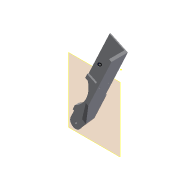
# Autodesk Inventor part: 30_CUBE_openSIM_Laserarm_532nm
Saved by Autodesk Inventor 2019 (Build 230136000, 136)
## iProperties
Created: 2019-08-28
Part Number: 30_CUBE_openSIM_Laserarm_532nm
Material: Generic
Document SubType Name: Modeling
Designer: diederichbenedict
Density: 1 g/cm^3
Appearance: Default
Author: diederichbenedict
Autodesk Inventor part; units mm, degrees
ref_plane "YZ Plane" through (0, 0, 0) normal (1, 0, 0) x (0, 1, 0)
ref_plane "Work Plane1" through (0, 0, 0) normal (0, 0, 1) x (1, 0, 0)
ref_plane "Work Plane3" through (52.5471, 38.1824, 4.95) normal (0, 0, -1) x (0, 1, 0)
sketch "Sketch1" plane through (0, 0, 0) normal (0, 0, 1) x (1, 0, 0)
  circle A0 centre (-41.7777, -39.8055) radius 1.9 projected
  circle A1 centre (-41.7777, -39.8055) radius 1.95
  line L0 (-60.1277, -15.7555) -> (-60.1277, 134.2445)
  line L1 (-41.7777, -39.8055) -> (3.034, 56.2936)
  line L2 (-41.7777, -39.8055) -> (64.2558, -39.8055) construction
  arc A2 (-52.0754, -35.9378) -> (-37.3201, -49.8618) centre (-41.7777, -39.8055) ccw construction
  circle A3 centre (-41.7777, -39.8055) radius 10
  line L3 (-50.8408, -35.5793) -> (-37.6025, -7.1896)
  line L4 (-32.6464, -43.882) -> (8.3579, 32.8366)
  line L5 (8.3579, 32.8366) -> (-14.0628, 43.2915)
  arc A4 (-37.6025, -7.1896) -> (-14.0628, 43.2915) centre (-56.4484, 32.3273) ccw
  line L6 (-14.0628, 43.2915) -> (8.0744, 90.7647)
  line L7 (8.3579, 32.8366) -> (-14.0628, 43.2915)
  line L8 (-14.0628, 43.2915) -> (10.4681, 95.8981)
  line L9 (10.4681, 95.8981) -> (32.8887, 85.4431)
  line L10 (32.8887, 85.4431) -> (8.3579, 32.8366)
  line L11 (12.5058, 41.7319) -> (32.8887, 85.4431) construction
  line L12 (-14.5928, 54.3682) -> (5.7901, 98.0794) projected
  line L13 (20.2457, 91.3387) -> (22.0583, 90.4934) construction
  line L14 (-14.0628, 43.2915) -> (-18.7407, 45.4729)
  line L15 (-18.7407, 45.4729) -> (5.7901, 98.0794)
  line L16 (5.7901, 98.0794) -> (10.4681, 95.8981)
  line L17 (10.4681, 95.8981) -> (-14.0628, 43.2915)
  point P0 (0, 0)
  dimension "d0" = 3.9
  dimension "d1" = 65
  dimension "d2" = 20
  constraints: 30 end point, 5 parallel, 4 point on circle, 3 centre point, 3 perpendicular, 2 coincident, 2 point on line, 2 tangent, 1 equal length, 1 horizontal, 1 vertical, 2 other
  measures "d0" diameter of A1
  measures "d1" angle of L2 L1
  measures "d2" diameter of A3
extrude "Extrusion1" add sketch "Sketch1" along normal up to surface (4.95 mm away) contours A3 L3 A4 L1 | L1 L5 L4 A3 | A3 | A4 L5 L1 | L5 L6 L8 L9 L10 | L14 L15 L12 L16 L8 L6
sketch "Sketch2" plane through (0, 0, 0) normal (0, 0, -1) x (-1, 0, 0)
  arc A0 (17.1277, 57.1088) -> (-27.3097, 31.2762) centre (46.6771, -44.8593) ccw projected
  arc A1 (17.4738, 55.9147) -> (-26.4433, 30.3846) centre (46.6771, -44.8593) ccw
  line L0 (17.4738, 55.9147) -> (17.4738, 109.5739)
  line L1 (17.4738, 109.5739) -> (-69.6922, 87.8202)
  line L2 (-69.6922, 87.8202) -> (-26.4433, 30.3846)
  point P0 (0, 0)
  constraints: 6 end point, 2 point on circle, 1 centre point, 1 vertical
ref_plane "Work Plane2" through (-67.0277, -18.5555, 3) normal (0, 0, 1) x (1, 0, 0)
extrude "Extrusion2" cut sketch "Sketch2" against normal up to surface (3 mm away)
sketch "Sketch3" plane through (-32.6464, -43.882, 10) normal (0.8819341, -0.4713727, 0) x (0, 0, -1)
  line L0 (10, 86.989) -> (5.05, 86.989) projected
  line L1 (10, 0) -> (5.05, 0) projected
  line L2 (10, 0) -> (10, 86.989) projected
  line L3 (10, 0) -> (10, 86.989) projected
  line L4 (10, -10.709) -> (5.05, -10.709) projected
  line L5 (5.05, 0) -> (5.05, 86.989) projected
  line L6 (7.525, -13.7861) -> (7.525, 7.904)
  line L7 (7.525, 7.904) -> (5.05, 12.7117)
  line L8 (5.05, -13.7861) -> (7.525, -13.7861)
  line L9 (10, -10.709) -> (5.05, -10.709) projected
  line L10 (5.05, -13.7861) -> (5.05, 12.7117)
  line L11 (10, -10.709) -> (5.05, -10.709) projected
  point P0 (10, 54.0897)
  point P1 (10, 95.7017)
  constraints: 8 end point, 1 parallel, 1 perpendicular, 1 point on line, 1 vertical
extrude "Extrusion3" cut sketch "Sketch3" along normal through all both and the other way through all contours L7 L6 L1 L5 | L6 L4 L10 L1 | L6 L8 L10 L4
sketch "Sketch4" plane through (10.4681, 95.8981, 4.95) normal (0.4226183, 0.9063078, 0) x (0.9063078, -0.4226183, 0)
  ellipse E0 centre (9.7884, -14.95) end of major axis (9.7884, -15.2253) minor radius 0.2495 projected
  circle A0 centre (9.7884, -14.95) radius 2.5581
  point P0 (31.041, 4.95)
  constraints: 1 centre point, 1 coincident, 1 other
sketch "Sketch5" plane through (-56.4484, 32.3273, 4.95) normal (0, 0, 1) x (0.9063078, -0.4226183, 0)
  arc A0 (53.1923, 7.7344) -> (52.9137, 5.7539) centre (53.053, 6.7442) ccw
  circle A1 centre (51.7192, 62.1648) radius 1.4
  circle A2 centre (35.4192, 62.1648) radius 1.4
  line L0 (33.7807, -45.188) -> (54.472, -46.3171)
  line L1 (54.472, -46.3171) -> (58.5192, 27.8499)
  line L2 (58.5192, 27.8499) -> (58.5192, 85.8948)
  line L3 (58.5192, 85.8948) -> (28.6192, 85.8948)
  line L4 (28.6192, 85.8948) -> (28.6192, 27.8499)
  line L5 (28.6192, 27.8499) -> (33.7807, 27.8499)
  arc A3 (33.7807, -27.8499) -> (33.7807, 27.8499) centre (0, 0) ccw
  line L6 (33.7807, -27.8499) -> (33.7807, -45.188)
  circle A4 centre (51.7192, 62.1648) radius 1.4
  circle A5 centre (35.4192, 62.1648) radius 1.4
  arc A6 (53.1923, 7.7344) -> (52.9137, 5.7539) centre (53.053, 6.7442) ccw
  circle A7 centre (53.053, 6.7442) radius 0.85
  line L7 (31.3609, 25.7869) -> (37.7001, 12.1923) construction
  line L8 (57.859, -31.0386) -> (37.7001, 12.1923) construction
  line L9 (31.524, -43.3188) -> (57.859, -31.0386) construction
  line L10 (32.8134, -60.0211) -> (31.524, -43.3188) construction
  arc A8 (32.8134, -60.0211) -> (52.0707, -66.4047) centre (43.7807, -59.1744) ccw construction
  line L11 (106.0309, -16.27) -> (52.0707, -66.4047) construction
  line L12 (103.5894, -11.0343) -> (106.0309, -16.27) construction
  line L13 (100.0207, -12.6984) -> (103.5894, -11.0343) construction
  arc A9 (98.0951, -13.5963) -> (100.0207, -12.6984) centre (98.5522, -12.063) ccw construction
  line L14 (97.6984, -13.7813) -> (98.0951, -13.5963) construction
  spline S0 degree 2 poles (96.5181, -11.2501) (96.4333, -12.0663) (96.3863, -12.5616) (96.3759, -12.7843) (96.416, -12.8869) (96.5684, -13.0113) (97.0261, -13.3267) (97.6984, -13.7813) knots 0 0 0 0.067676 0.185094 0.471221 0.770579 0.933711 1 1 1 weights 1.003789 1.886908 3.975326 7.291888 7.731646 4.465678 1.868813 1.003789 construction
  line L15 (97.7807, -10.6613) -> (96.5181, -11.2501) construction
  line L16 (102.4091, -8.5031) -> (97.9745, -10.571) construction
  line L17 (83.7226, 31.5703) -> (102.4091, -8.5031) construction
  arc A10 (83.7226, 31.5703) -> (79.0045, 33.4837) centre (41.4762, -65.8253) ccw construction
  arc A11 (76.3548, 34.4451) -> (79.0045, 33.4837) centre (77.4213, 33.2524) ccw construction
  arc A12 (76.3548, 34.4451) -> (25.1635, 39.0773) centre (41.4762, -65.8253) ccw construction
  line L18 (31.3609, 25.7869) -> (25.1635, 39.0773) construction
  arc A13 (53.1923, 7.7344) -> (52.9137, 5.7539) centre (53.053, 6.7442) ccw construction
  arc A14 (83.5786, -4.5713) -> (53.1923, 7.7344) centre (43.7807, -59.1744) ccw construction
  arc A15 (82.4006, -6.1875) -> (83.5786, -4.5713) centre (82.9896, -5.3794) ccw construction
  arc A16 (82.4006, -6.1875) -> (52.9137, 5.7539) centre (43.7807, -59.1744) ccw construction
  circle A17 centre (43.7807, -59.1744) radius 1.9 construction
  circle A18 centre (94.3261, -2.9999) radius 1.6 construction
  circle A19 centre (62.4812, -28.8832) radius 1.4 construction
  circle A20 centre (55.6561, 6.308) radius 0.879
  circle A21 centre (50.3192, 7.1869) radius 0.879
  arc A22 (97.9745, -10.571) -> (97.7807, -10.6613) centre (98.5522, -12.063) ccw
  point P0 (64.8217, -5.4424)
  dimension "d14" = 1.7
  constraints: 3 centre point, 1 coincident
  measures "d14" diameter of A7
extrude "Extrusion4" cut sketch "Sketch5" against normal blind 10 contours A1 | A2 | A7 | A20 | A21
sketch "Sketch6" plane through (-56.4484, 32.3273, 4.95) normal (0, 0, 1) x (0.9063078, -0.4226183, 0)
  circle A0 centre (53.053, 6.7442) radius 0.85 projected
  line L0 (33.7807, -45.188) -> (54.472, -46.3171) projected
  line L1 (54.472, -46.3171) -> (58.5192, 27.8499) projected
  line L2 (58.5192, 27.8499) -> (58.5192, 85.8948) construction
  line L3 (58.5192, 85.8948) -> (28.6192, 85.8948) projected
  line L4 (28.6192, 85.8948) -> (28.6192, 27.8499) projected
  line L5 (28.6192, 27.8499) -> (33.7807, 27.8499) projected
  arc A1 (33.7807, -27.8499) -> (33.7807, 27.8499) centre (0, 0) ccw projected
  line L6 (33.7807, -27.8499) -> (33.7807, -45.188) projected
  line L7 (28.6192, 38.3041) -> (28.6192, 27.8499) projected
  line L8 (28.6192, 36.406) -> (58.5192, 36.406)
  line L9 (58.5192, 27.8499) -> (58.5192, 85.8948) projected
  arc A2 (58.5192, 37.7014) -> (28.6192, 38.3041) centre (41.4762, -65.8253) ccw projected
  line L10 (50.5692, 37.6648) -> (56.5192, 37.6648) projected
  point P0 (64.8217, -5.4424)
  constraints: 2 coincident, 2 end point, 2 point on line, 1 perpendicular
extrude "Extrusion5" add sketch "Sketch6" along normal blind 3 contours L6 A1 L5 L4 L8 L9 L1 L0
sketch "Sketch7" plane through (12.5213, 41.7651, 3) normal (0.9063078, -0.4226183, 0) x (0, 0, -1)
  line L0 (0, 0) -> (0, 48.1934) projected
  line L1 (0, 48.1934) -> (-1.95, 48.1934) projected
  line L2 (-1.95, -1.2954) -> (-1.95, 48.1934) projected
  line L3 (-1.95, -1.2954) -> (-4.95, -1.2954) projected
  line L4 (-4.95, -9.8515) -> (-4.95, -1.2954) projected
  line L5 (3, -9.8515) -> (-4.95, -9.8515) projected
  line L6 (3, -9.8515) -> (3, 0) projected
  line L7 (3, 0) -> (0, 0) projected
  arc A0 (-23.9, 25.2618) -> (-23.9, 23.665) centre (-25.05, 24.4634) ccw projected
  arc A1 (-9.9, 23.665) -> (-9.9, 25.2618) centre (-8.75, 24.4634) ccw projected
  line L8 (0.525, -88.819) -> (0.525, -96.7113) projected
  line L9 (3, -96.7113) -> (0.525, -96.7113) projected
  line L10 (3, -96.7113) -> (3, -9.8515) projected
  line L11 (3, -9.8515) -> (-4.95, -9.8515) projected
  line L12 (-4.95, -84.0185) -> (-4.95, -9.8515) projected
  line L13 (-1.95, -84.0185) -> (-4.95, -84.0185) projected
  line L14 (-1.95, -84.0185) -> (0.525, -88.819) projected
  line L15 (0, 48.1934) -> (-1.95, 48.1934) projected
  line L16 (0, 48.1934) -> (-30, 48.1934)
  line L17 (-30, 48.1934) -> (-30, -11.8066)
  line L18 (-30, -11.8066) -> (0, -11.8066)
  line L19 (0, -11.8066) -> (0, 48.1934)
  circle A2 centre (-8.75, 24.4634) radius 1.4
  circle A3 centre (-25.05, 24.4634) radius 1.4
  point P0 (3, -43.1438)
  dimension "d17" = 30
  dimension "d18" = 60
  dimension "d19" = 2.8
  dimension "d20" = 2.8
  constraints: 8 end point, 2 centre point, 2 coincident, 2 parallel, 1 horizontal, 1 perpendicular
  measures "d17" distance of L18.end L17.end
  measures "d18" distance of L17.end L16.end
  measures "d19" diameter of A2
  measures "d20" diameter of A3
extrude "Extrusion6" add sketch "Sketch7" along normal blind 5 contours L19 L5 L4 L3 L2 L1 L0 | L19 L18 L12 L5 | L2 L3 L4 L12 L18 L17 L16
sketch "Sketch8" plane through (-32.6464, -43.882, 2.475) normal (0.8819341, -0.4713727, 0) x (0, 0, -1)
  line L0 (0, 7.904) -> (0, 0) projected
  line L1 (2.475, 0) -> (0, 0) projected
  line L2 (2.475, 0) -> (2.475, 86.989) projected
  line L3 (2.475, 86.989) -> (-0.525, 86.989) projected
  line L4 (-0.525, 86.989) -> (-5.475, 86.989) projected
  line L5 (-5.475, 12.7117) -> (-5.475, 86.989) projected
  line L6 (-2.475, 12.7117) -> (-5.475, 12.7117) projected
  line L7 (-2.475, 12.7117) -> (0, 7.904) projected
  line L8 (-30.525, 85.0369) -> (-0.525, 85.0369) projected
  line L9 (-30.525, 85.0369) -> (-5.475, 12.7117)
  line L10 (-30.525, 85.0369) -> (2.475, 85.0369)
  line L11 (2.475, 85.0369) -> (2.475, 86.989)
  line L12 (2.475, 86.989) -> (-30.525, 86.989)
  line L13 (-30.525, 86.989) -> (-30.525, 85.0369)
  point P0 (2.475, 54.0897)
  constraints: 10 end point, 2 parallel, 1 horizontal, 1 perpendicular
extrude "Extrusion7" add sketch "Sketch8" along normal blind 5
sketch "Sketch9" plane through (17.0529, 39.652, 3) normal (0.9063078, -0.4226183, 0) x (0, 0, -1)
  line L0 (1.134, -64.339) -> (-34.934, -64.339) projected
  line L1 (-30, -11.8066) -> (0, -11.8066) projected
  line L2 (-30, -11.8066) -> (-30, -12.0732) projected
  line L3 (-30, -12.0732) -> (-4.95, -84.291) projected
  line L4 (-4.95, -84.291) -> (-1.95, -84.291) projected
  line L5 (-1.95, -84.291) -> (0.525, -89.0915) projected
  line L6 (0.525, -89.0915) -> (0.525, -96.9838) projected
  line L7 (0.525, -96.9838) -> (3, -96.9838) projected
  line L8 (3, -96.9838) -> (3, -10.124) projected
  line L9 (3, -10.124) -> (0, -10.124) projected
  line L10 (0, -11.8066) -> (0, -10.124) projected
  line L11 (0, -11.8066) -> (0, -10.124) projected
  line L12 (-30, -12.0732) -> (0, -12.0732)
  line L13 (0, -12.0732) -> (0, -10.124)
  line L14 (0, -10.124) -> (-30, -10.124)
  line L15 (-30, -10.124) -> (-30, -12.0732)
  point P0 (3, -43.1438)
  constraints: 8 end point, 2 parallel, 1 horizontal, 1 perpendicular
extrude "Extrusion8" add sketch "Sketch9" along normal up to surface surface through (-5.0485, -2.8539, 10.3013) normal (0.8819341, -0.4713727, 0)
sketch "Sketch10" plane through (-50.8408, -35.5793, 2.475) normal (0, 0, 1) x (0.9063078, -0.4226183, 0)
  arc A0 (-18.3686, 9.3717) -> (-15.3461, 9.752) centre (-16.7962, 9.0758) ccw construction
  line L0 (-21.8064, 16.7441) -> (-18.3686, 9.3717) construction
  arc A1 (-22.5948, 18.4348) -> (-21.8064, 16.7441) centre (-21.0224, 18.1389) ccw construction
  line L1 (-38.1333, 51.7573) -> (-22.5948, 18.4348) construction
  line L2 (-38.1333, 51.7573) -> (-41.2527, 50.3026) construction
  line L3 (-41.2527, 50.3026) -> (-47.592, 63.8973) construction
  line L4 (-47.592, 63.8973) -> (-44.4725, 65.3519) construction
  line L5 (-59.2642, 97.0726) -> (-44.4725, 65.3519) construction
  line L6 (-59.2642, 97.0726) -> (-62.3836, 95.618) construction
  line L7 (-62.3836, 95.618) -> (-68.7229, 109.2126) construction
  line L8 (-68.7229, 109.2126) -> (-65.6035, 110.6673) construction
  line L9 (-80.0993, 141.7536) -> (-65.6035, 110.6673) construction
  line L10 (-80.0993, 141.7536) -> (-38.0466, 161.3631) construction
  line L11 (-38.0466, 161.3631) -> (-23.5508, 130.2767) construction
  line L12 (-23.5508, 130.2767) -> (-17.2115, 116.6821) construction
  line L13 (-17.2115, 116.6821) -> (-8.6173, 98.2517) construction
  arc A2 (42.5741, 93.6195) -> (-8.6173, 98.2517) centre (7.6955, -6.6509) ccw construction
  arc A3 (45.2238, 92.6582) -> (42.5741, 93.6195) centre (43.6406, 92.4268) ccw construction
  arc A4 (49.9419, 90.7447) -> (45.2238, 92.6582) centre (7.6955, -6.6509) ccw construction
  line L14 (49.9419, 90.7447) -> (4.6425, 187.8896) construction
  arc A5 (4.6425, 187.8896) -> (1.9846, 188.857) centre (2.8298, 187.0444) ccw construction
  line L15 (1.9846, 188.857) -> (-84.8397, 148.3701) construction
  arc A6 (-84.8397, 148.3701) -> (-85.8071, 145.7123) centre (-83.9944, 146.5575) ccw construction
  line L16 (-85.8071, 145.7123) -> (-3.0584, -31.7428) construction
  arc A7 (-3.0584, -31.7428) -> (-0.4005, -32.7101) centre (-1.2458, -30.8975) ccw construction
  line L17 (-0.4005, -32.7101) -> (86.4237, 7.7767) construction
  arc A8 (86.4237, 7.7767) -> (87.3911, 10.4345) centre (85.5785, 9.5893) ccw construction
  line L18 (87.3911, 10.4345) -> (72.2501, 42.9045) construction
  line L19 (72.2501, 42.9045) -> (18.2899, -7.2303) construction
  arc A9 (-0.9674, -0.8466) -> (18.2899, -7.2303) centre (10, 0) ccw construction
  line L20 (-0.9674, -0.8466) -> (-2.2567, 15.8556) construction
  line L21 (-2.2567, 15.8556) -> (-15.3461, 9.752) construction
  circle A10 centre (-43.9366, 161.9267) radius 1.6 construction
  circle A11 centre (1.3788, 183.0576) radius 1.6 construction
  circle A12 centre (22.5097, 137.7422) radius 1.6 construction
  circle A13 centre (45.4239, -6.0456) radius 1.6 construction
  circle A14 centre (-80.1889, 145.0219) radius 1.6 construction
  circle A15 centre (81.5917, 11.0404) radius 1.6 construction
  circle A16 centre (0.2053, -26.9108) radius 1.6 construction
  circle A17 centre (36.3609, -10.2718) radius 1.6 construction
  circle A18 centre (39.4144, 101.4899) radius 1.6 construction
  circle A19 centre (18.2835, 146.8053) radius 1.6 construction
  circle A20 centre (-34.8735, 166.1529) radius 1.6 construction
  arc A21 (0, 0) -> (19.9986, 0.1645) centre (10, 0) ccw construction
  line L22 (19.9986, 0.1645) -> (29.7384, 33.2112)
  line L23 (29.7384, -0.108) -> (29.7384, 86.7519) projected
  arc A22 (0, 0) -> (19.9986, 0.1645) centre (10, 0) ccw projected
  line L24 (19.9986, 0.1645) -> (22.5097, -3.3097)
  line L25 (31.7799, -3.9815) -> (22.5097, -3.3097)
  line L26 (31.7799, -3.9815) -> (29.7384, 33.2112)
  point P0 (31.041, 53.7321)
  constraints: 8 end point, 2 point on line
extrude "Extrusion9" cut sketch "Sketch10" along normal through all both and the other way through all
sketch "Sketch11" plane through (-50.8408, -35.5793, 0) normal (-0.9063078, 0.4226183, 0) x (0, 0, 1)
  line L0 (2.475, 0) -> (2.475, 9.1716) projected
  line L1 (2.475, 9.1716) -> (4.95, 13.9864) projected
  line L2 (4.95, 13.9864) -> (7.95, 13.9864) projected
  line L3 (7.95, 31.3246) -> (7.95, 13.9864) projected
  line L4 (0, 31.3246) -> (7.95, 31.3246) projected
  line L5 (0, 31.3246) -> (0, 0) projected
  line L6 (0, 0) -> (2.475, 0) projected
  line L7 (2.475, 0) -> (2.475, 9.1716) projected
  line L8 (2.475, 9.1716) -> (2.475, 16.6568)
  line L9 (2.475, 16.6568) -> (7.95, 22.1749)
  line L10 (7.95, 22.1749) -> (14.3557, 31.3246)
  line L11 (33, 85.075) -> (7.95, 12.8573) projected
  line L12 (0, 31.3246) -> (7.95, 31.3246) projected
  line L13 (7.95, 31.3246) -> (14.3557, 31.3246)
  line L14 (2.475, 9.1716) -> (4.95, 13.9864) projected
  line L15 (2.475, 9.1716) -> (12.1097, 9.1716)
  line L16 (12.1097, 9.1716) -> (14.3557, 31.3246)
  line L17 (2.475, 9.1716) -> (11.7622, 9.1716)
  line L18 (11.7622, 9.1716) -> (11.7622, 5.7438)
  line L19 (11.7622, 5.7438) -> (2.475, 5.7438)
  line L20 (2.475, 5.7438) -> (2.475, 9.1716)
  point P0 (0, 53.7321)
  constraints: 20 end point, 3 point on line, 2 horizontal, 2 parallel, 1 collinear, 1 perpendicular
extrude "Extrusion10" cut sketch "Sketch11" against normal through all contours L0 L15 L18 L19 | L8 L9 L3 L2 L1 | L1 L2 L3 L10 L16 L15
sketch "Sketch12" plane through (5.7901, 98.0794, 4.95) normal (0.4226183, 0.9063078, 0) x (0.9063078, -0.4226183, 0)
  line L0 (34.9, 1.95) -> (0, 1.95) projected
  line L1 (0, 1.95) -> (0, 0) projected
  line L2 (29.9, 0) -> (0, 0) projected
  line L3 (29.9, 0) -> (29.9, -28.05) projected
  line L4 (29.9, -28.05) -> (34.9, -28.05) projected
  line L5 (34.9, 1.95) -> (34.9, -28.05) projected
  point P0 (36.2025, 4.95)
extrude "Extrusion11" add sketch "Sketch12" along normal blind 40
body "Solid1"
